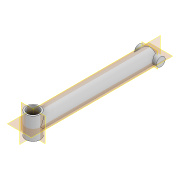
# Autodesk Inventor part: LowerlegP
Saved by Autodesk Inventor 2021 (Build 250183000, 183)
## iProperties
Created: 2020-12-19
Part Number: LowerlegP
Material: 一般
Document SubType Name: Modeling
Designer: Tazaki
Density: 1.80077 g/cm^3
Appearance: 既定
Mass: 1500 g
Surface Area: 866.22 cm^2
Volume: 832.978 cm^3
Author: Tazaki
Autodesk Inventor part; units mm, degrees
ref_plane "作業平面1" through (0, 0, -400) normal (0, 0, 1) x (1, 0, 0)
sketch "スケッチ3" plane through (0, 0, 0) normal (0, 0, 1) x (1, 0, 0)
  circle A0 centre (0, 0) radius 25
  dimension "d7" = 50
  constraints: 1 centre point, 1 coincident
  measures "d7" diameter of A0
extrude "押し出し2" add sketch "スケッチ3" against normal blind 400
sketch "スケッチ4" plane through (0, 0, 0) normal (0, 1, 0) x (-1, 0, 0)
  circle A0 centre (0, 0) radius 25
  dimension "d10" = 50
  constraints: 1 centre point, 1 coincident
  measures "d10" diameter of A0
extrude "押し出し3" add sketch "スケッチ4" along normal mid plane 75
sketch "スケッチ5" plane through (0, -37.5, 0) normal (0, -1, 0) x (1, 0, 0)
  circle A0 centre (0, 0) radius 20
  dimension "d13" = 40
  constraints: 1 centre point, 1 coincident
  measures "d13" diameter of A0
extrude "押し出し4" cut sketch "スケッチ5" against normal blind 75
sketch "スケッチ6" plane through (0, 0, 0) normal (1, 0, 0) x (0, 1, 0)
  circle A0 centre (0, -400) radius 15
  line L0 (-52.5, 0) -> (52.5, 0) projected
  point P0 (0, 0)
  dimension "d16" = 30
  dimension "d17" = 400
  constraints: 1 centre point, 1 vertical alignment
  measures "d16" diameter of A0
  measures "d17" distance from line of L0 A0.centre
extrude "押し出し5" add sketch "スケッチ6" along normal mid plane 75
